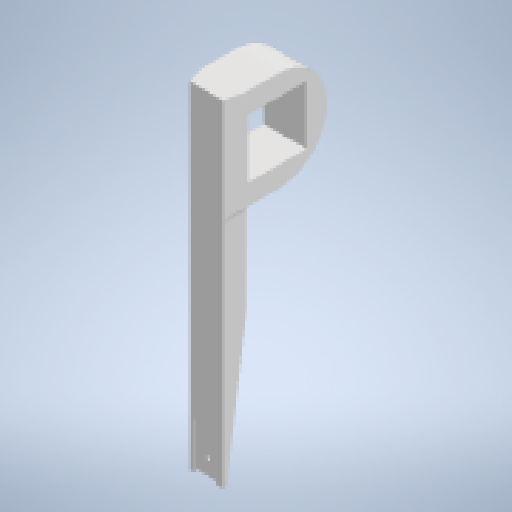
# Autodesk Inventor part: washing_arm
Saved by Autodesk Inventor 2023.3 (Build 273359000, 359)
## iProperties
Created: 2023-11-21
Part Number: washing_arm
Material: Generic
Document SubType Name: Modeling
Designer: mmelin
Density: 1 g/cm^3
Appearance: Default
Author: mmelin
Autodesk Inventor part; units mm, degrees
ref_plane "YZ Plane" through (0, 0, 0) normal (1, 0, 0) x (0, 1, 0)
ref_plane "XZ Plane" through (0, 0, 0) normal (0, 1, 0) x (-1, 0, 0)
ref_plane "XY Plane" through (0, 0, 0) normal (0, 0, 1) x (1, 0, 0)
sketch "Sketch1" plane through (0, 0, 0) normal (1, 0, 0) x (0, 1, 0)
  circle A0 centre (0, 0) radius 6.604
  circle A1 centre (0, 0) radius 10.604
  line L0 (10.604, 0) -> (-10.604, 0)
  line L1 (-10.604, 0) -> (-10.604, 10.604)
  line L2 (-10.604, 10.604) -> (10.604, 10.604)
  line L3 (10.604, 10.604) -> (10.604, 0)
  line L4 (0.9188, 26.2008) -> (13.3268, 26.2008) projected
  line L5 (13.3268, 26.2008) -> (13.3268, 13.7928) projected
  line L6 (13.3268, 13.7928) -> (0.9188, 13.7928) projected
  line L7 (0.9188, 13.7928) -> (0.9188, 26.2008) projected
  line L8 (6.204, 6.204) -> (-6.204, 6.204)
  line L9 (-6.204, 6.204) -> (-6.204, -6.204)
  line L10 (-6.204, -6.204) -> (6.204, -6.204)
  line L11 (6.204, -6.204) -> (6.204, 6.204)
  line L12 (6.204, 6.204) -> (-6.204, -6.204) construction
  line L13 (-6.204, 6.204) -> (6.204, -6.204) construction
  point P0 (-10.604, 0)
  point P1 (0, 10.604)
  dimension "d1" = 21.208
  dimension "d0" = 13.208
  constraints: 20 end point, 6 parallel, 3 horizontal, 2 coincident, 2 midpoint, 2 perpendicular, 2 vertical, 1 centre point, 3 other
  measures "d0" diameter of A0
extrude "Extrusion1" add sketch "Sketch1" along normal blind 9 contours L0 L11 A0 | L0 A1 A0 L9 L10 L11 | A0 L11 L8 L9 L0 A1 | A0 L11 L0 | A1 L2 L3 | L8 A0 | A0 L10 | L1 L2 A1 | L9 A0 L0 | L0 A0 L9
sketch "Sketch2" plane through (0, -10.604, 0) normal (0, -1, 0) x (1, 0, 0)
  line L0 (0, 0) -> (0, 10.604) projected
  line L1 (9, 0) -> (9, 10.604) projected
  line L2 (1, 10.604) -> (8, 10.604)
  line L3 (8, 10.604) -> (8, 5.604)
  line L4 (8, 5.604) -> (1, 5.604)
  line L5 (1, 5.604) -> (1, 10.604)
  line L6 (0, 10.604) -> (9, 10.604) projected
  dimension "d16" = 1
  dimension "d17" = 1
  dimension "d18" = 5
  constraints: 8 end point, 2 parallel, 1 collinear, 1 horizontal, 1 perpendicular
  measures "d16" distance between parallel lines of L1 L3
  measures "d17" distance between parallel lines of L0 L5
  measures "d18" distance between parallel lines of L2 L4
extrude "Extrusion2" add sketch "Sketch2" along normal blind 50
sketch "Sketch3" plane through (0, -60.604, 0) normal (0, -1, 0) x (1, 0, 0)
  line L0 (1.8687, 9.964) -> (7.1313, 9.964)
  line L1 (1.8687, 9.964) -> (2.2382, 10.604)
  line L2 (7.1313, 9.964) -> (6.7618, 10.604)
  line L3 (1.8687, 9.964) -> (2.7375, 9.964) construction
  line L4 (7.1313, 9.964) -> (8, 9.964) construction
  line L5 (8, 10.604) -> (1, 10.604) projected
  line L6 (1.8687, 9.964) -> (1, 9.964) construction
  line L7 (1, 10.604) -> (1, 5.604) construction
  line L8 (8, 5.604) -> (8, 10.604) construction
  point P0 (0, 0)
  dimension "d7" = 60
  dimension "d8" = 60
  dimension "d19" = 0.64
  dimension "d51" = 4.5235
  constraints: 12 end point, 4 point on line, 3 equal length, 2 horizontal, 1 collinear
  measures "d7" angle of L0 L1
  measures "d8" angle of L0 L2
  measures "d19" distance between parallel lines of L5 L0
  measures "d51" distance of L2.end L1.end
extrude "Extrusion3" cut sketch "Sketch3" against normal blind 10
chamfer "Chamfer1" distance 4 distance2 30 1 edges at (4.5, -60.604, 5.604) measured on face at (4.5, -60.604, 6.104)
sketch "Sketch4" plane through (1.8687, -60.604, 9.964) normal (0, 0, 1) x (1, 0, 0)
  circle A0 centre (2.6313, 3.5) radius 0.45
  line L0 (2.6313, 3.5) -> (6.1313, 3.5) construction
  line L1 (2.6313, 3.5) -> (-0.8687, 3.5)
  line L2 (-0.8687, 50) -> (-0.8687, 0) construction
  line L3 (6.1313, 50) -> (6.1313, 0) construction
  line L4 (5.2625, 0) -> (0, 0) construction
  point P0 (-1.8687, 60.604)
  point P1 (-0.329, 47)
  point P2 (2.671, 47)
  dimension "d21" = 0.9
  dimension "d22" = 3.5
  constraints: 4 end point, 3 horizontal, 1 centre point, 1 collinear, 4 other
  measures "d21" diameter of A0
  measures "d22" distance from line of L4 L0.start
extrude "Extrusion4" cut sketch "Sketch4" against normal blind 10
sketch "Sketch5" plane through (1.8687, -60.604, 9.964) normal (0, 0, 1) x (1, 0, 0)
  circle A0 centre (2.6313, 3.5) radius 0.45 projected
  circle A1 centre (2.6313, 3.5) radius 0.75
  point P0 (-1.8687, 60.604)
  dimension "d25" = 1.5
  constraints: 1 centre point, 1 coincident
  measures "d25" diameter of A1
extrude "Extrusion5" add sketch "Sketch5" against normal blind 1.5
chamfer "Chamfer2" distance 1.5 distance2 9 2 edges at (0, 0, 10.604) (9, 0, 10.604) measured on face at (8.5, 0, 10.604) measured on face at (0.5, 0, 10.604)
ref_plane "Work Plane1" through (4.5, 0, 0) normal (-1, 0, 0) x (0, 0, 1)
ref_plane "Work Plane2" through (0, 10.604, 0) normal (0, 1, 0) x (-1, 0, 0)
fillet "Fillet2" radius 2 2 edges at (1, -10.604, 6.604) (8, -10.604, 6.604)
ref_plane "Work Plane3" through (4.5, 0, 0) normal (1, 0, 0) x (0, 0, -1)
chamfer "Chamfer3" distance 0.2 angle 45 3 edges at (4.5, -60.604, 9.964) (2.0535, -60.604, 10.284) (6.9465, -60.604, 10.284)
equation "\"d17\" = d16"
equation "\"d8\" = d7"
body "Solid1"
